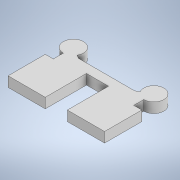
# Autodesk Inventor part: ZTopSpacer
Saved by Autodesk Inventor 2020 (Build 240168000, 168)
## iProperties
Created: 2022-06-05
Part Number: ZTopSpacer
Material: Ogólny
Document SubType Name: Modeling
Designer: mikoma
Density: 1 g/cm^3
Appearance: Domyślna
Author: mikoma
Autodesk Inventor part; units mm, degrees
ref_plane "YZ Plane" through (0, 0, 0) normal (1, 0, 0) x (0, 1, 0)
ref_plane "XZ Plane" through (0, 0, 0) normal (0, 1, 0) x (-1, 0, 0)
ref_plane "XY Plane" through (0, 0, 0) normal (0, 0, 1) x (1, 0, 0)
sketch "Szkic1" plane through (0, 0, 0) normal (0, 1, 0) x (-1, 0, 0)
  arc A0 (-21, -3.0839) -> (-14.3876, -6.8785) centre (-20, -9) ccw
  line L0 (-21, 0) -> (-21, -3.0839)
  line L1 (-25, 0) -> (-21, 0)
  line L2 (-25, 20.5) -> (-25, 0)
  line L3 (-4.5, 20.5) -> (-25, 20.5)
  line L4 (-4.5, 0) -> (-4.5, 20.5)
  line L5 (4.5, 0) -> (-4.5, 0)
  line L6 (4.5, 20.5) -> (4.5, 0)
  line L7 (25, 20.5) -> (4.5, 20.5)
  line L8 (25, 0) -> (25, 20.5)
  line L9 (21, 0) -> (25, 0)
  line L10 (21, -3.0839) -> (21, 0)
  arc A1 (14.3876, -6.8785) -> (21, -3.0839) centre (20, -9) ccw
  line L11 (13.7321, -6.5) -> (14.3876, -6.8785)
  line L12 (-13.7321, -6.5) -> (13.7321, -6.5)
  line L13 (-14.3876, -6.8785) -> (-13.7321, -6.5)
  point P0 (0, 0)
  point P1 (0, 0)
  dimension "d0" = 9
  dimension "d1" = 50
  dimension "d2" = 6
  dimension "d3" = 150
  dimension "d4" = 150
  dimension "d5" = 9
  dimension "d6" = 20
  dimension "d7" = 20
  dimension "d8" = 20.5
  dimension "d9" = 6.5
  dimension "d10" = 4
  dimension "d11" = 9
  dimension "d12" = 0.6555
  constraints: 28 end point, 8 perpendicular, 6 equal length, 4 point on circle, 2 centre point, 2 horizontal, 1 equal radius, 1 horizontal alignment, 1 midpoint
  measures "d0" distance between parallel lines of L4 L6
  measures "d1" distance between parallel lines of L2 L8
  measures "d2" radius of A1
  measures "d3" angle of L11 L12
  measures "d4" angle of L12 L13
  measures "d5" distance from line of L5 A1.centre
  measures "d6" horizontal distance of A1.centre point (0, 0)
  measures "d7" horizontal distance of A0.centre point (0, 0)
  measures "d8" distance between parallel lines of L5 L7
  measures "d9" distance between parallel lines of L5 L12
  measures "d10" distance of L9.start L9.end
  measures "d11" distance from line of L9 A1.centre
  measures "d12" horizontal distance of L12.end L11.end
extrude "Wyciągnięcie proste1" add sketch "Szkic1" along normal blind 5
thicken "Pogrubienie2" operation add thickness 1 both sides no extend neighbours yes toward (0, 0, -1) faces at (11.3333, 1.6667, 20.5) (25, 3.3333, 13.6667) (23.6667, 1.6667, 0) (21, 1.6667, -1.028) (24.3935, 3.3333, -4.9138) (14.1691, 1.6667, -6.7523) (4.5774, 1.6667, -6.5) (-13.9506, 1.6667, -6.6262) (-18.2455, 3.3333, -14.7377) (-21, 1.6667, -2.0559) (-22.3333, 1.6667, 0) (-25, 1.6667, 6.8333) (-18.1667, 3.3333, 20.5) (-4.5, 3.3333, 13.6667) (-1.5, 1.6667, 0) (4.5, 3.3333, 6.8333)
